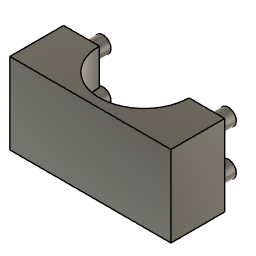
dpv2_cover (Autodesk Fusion 360 design; units mm, degrees)
Autodesk Fusion 360 part; units mm, degrees
note: some values were not read from the file. Set by a fixed rule: which face or edge a step refers to.
sketch "スケッチ1" plane through (0, 0, 0) normal (0, 1, 0) x (1, 0, 0)
  line L0 (-21, 0) -> (21, 0)
  line L1 (21, 0) -> (21, -72.5)
  line L2 (21, -72.5) -> (-21, -72.5)
  line L3 (-21, -72.5) -> (-21, 0)
  line L4 (6.5, -72.5) -> (-6.5, -72.5)
  line L5 (-6.5, -72.5) -> (-6.5, -96.5)
  line L6 (-6.5, -96.5) -> (6.5, -96.5)
  line L7 (6.5, -96.5) -> (6.5, -72.5)
  line L8 (-12.5, -160.5) -> (9, -160.5)
  line L9 (9, -160.5) -> (9, -96.5)
  line L10 (9, -96.5) -> (-12.5, -96.5)
  line L11 (-12.5, -96.5) -> (-12.5, -160.5)
  line L12 (-21, -67.5) -> (21, -67.5) construction
  circle A0 centre (-12, -67.5) radius 1.75
  circle A1 centre (12, -67.5) radius 1.75
  line L13 (0, -1.75) -> (0, -22.5)
  circle A2 centre (0, -155.5) radius 2
  dimension "d1" = 42
  dimension "d2" = 5
  dimension "d3" = 3.5
  dimension "d4" = 3.5
  dimension "d5" = 24
  dimension "d6" = 72.5
  dimension "d7" = 13
  dimension "d8" = 2.5
  dimension "d9" = 6
  dimension "d10" = 24
  dimension "d11" = 64
  dimension "d12" = 4
  dimension "d13" = 5
  constraint horizontal L0
  constraint vertical L1
  constraint horizontal L2
  constraint vertical L3
  constraint horizontal L4
  constraint vertical L5
  constraint horizontal L6
  constraint vertical L7
  constraint coincident L2 L4.start
  constraint horizontal L8
  constraint vertical L9
  constraint horizontal L10
  constraint vertical L11
  constraint midpoint origin L0
  constraint coincident L3 L12.start
  constraint coincident L1 L12.end
  constraint perpendicular L1 L12
  constraint coincident L12 A0.centre
  constraint coincident L12 A1.centre
  constraint symmetric A0 A1 L13
  constraint symmetric L5 L7 L13
  constraint coincident L13 A2.centre
  measures "d1" distance of L0.start L0.end
  measures "d2" distance of L2 L12
  measures "d3" diameter of A0
  measures "d4" diameter of A1
  measures "d5" distance of A0.centre A1.centre
  measures "d6" distance of L0.start L2.end
  measures "d7" distance of L5.end L6.end
  measures "d8" distance of L6.end L9.end
  measures "d9" distance of L5.end L10.end
  measures "d10" distance of L4.end L5.end
  measures "d11" distance of L8.start L10.end
  measures "d12" diameter of A2
  measures "d13" distance of L8 A2.centre
extrude "押し出し1" add sketch "スケッチ1" against normal blind 2 makes body 1
sketch "スケッチ2" plane through (0, 0, 0) normal (0, 1, 0) x (-1, 0, 0)
  circle A0 centre (12, 67.5) radius 1.75
  circle A1 centre (-12, 67.5) radius 1.75
  circle A2 centre (0, 155.5) radius 2
  line L0 (6.5, 72.5) -> (6.5, 96.5)
  line L1 (6.5, 96.5) -> (12.5, 96.5)
  line L2 (12.5, 96.5) -> (12.5, 160.5)
  line L3 (12.5, 160.5) -> (-9, 160.5)
  line L4 (-9, 160.5) -> (-9, 96.5)
  line L5 (-9, 96.5) -> (-6.5, 96.5)
  line L6 (-6.5, 96.5) -> (-6.5, 72.5)
  line L7 (-6.5, 72.5) -> (-21, 72.5)
  line L8 (-21, 72.5) -> (-21, 0)
  line L9 (-21, 0) -> (21, 0)
  line L10 (21, 0) -> (21, 72.5)
  line L11 (21, 72.5) -> (6.5, 72.5)
  line L12 (-21, 0) -> (-22.5, 0)
  line L13 (-22.5, 0) -> (-22.5, 74)
  line L14 (-22.5, 74) -> (-8, 74)
  line L15 (-8, 74) -> (-8, 95)
  line L16 (-8, 95) -> (-10.5, 95)
  line L17 (-10.5, 95) -> (-10.5, 160.5)
  line L18 (-10.5, 160.5) -> (-9, 160.5)
  line L19 (12.5, 160.5) -> (14, 160.5)
  line L20 (14, 160.5) -> (14, 95)
  line L21 (14, 95) -> (8, 95)
  line L22 (8, 95) -> (8, 74)
  line L23 (8, 74) -> (22.5, 74)
  line L24 (22.5, 74) -> (22.5, 0)
  line L25 (22.5, 0) -> (21, 0)
  dimension "d16" = 1.5
  dimension "d17" = 1.5
  dimension "d18" = 1.5
  dimension "d19" = 1.5
  dimension "d20" = 1.5
  dimension "d22" = 1.5
  dimension "d23" = 1.5
  dimension "d24" = 1.5
  dimension "d25" = 1.5
  dimension "d26" = 1.5
  constraint coincident L8.end L9.start
  constraint perpendicular L8 L12
  constraint perpendicular L9 L13
  constraint perpendicular L13 L14
  constraint perpendicular L14 L15
  constraint perpendicular L15 L16
  constraint perpendicular L16 L17
  constraint coincident L3.end L4.start
  constraint coincident L2.end L3.start
  constraint perpendicular L2 L19
  constraint perpendicular L3 L20
  constraint perpendicular L0 L21
  constraint perpendicular L3 L22
  constraint perpendicular L0 L23
  constraint perpendicular L3 L24
  constraint coincident L9.end L10.start
  constraint perpendicular L24 L25
  constraint perpendicular L17 L18
  measures "d16" distance of L2.end L19.end
  measures "d17" distance of L17.end L3.end
  measures "d18" distance of L6 L15
  measures "d19" distance of L5 L16
  measures "d20" distance of L7 L14
  measures "d22" distance of L8.end L12.end
  measures "d23" distance of L24.end L9.end
  measures "d24" distance of L11 L23
  measures "d25" distance of L0 L22
  measures "d26" distance of L1 L21
extrude "押し出し2" add sketch "スケッチ2" against normal blind 15 contours L0 L1 L2 L10 L11 L19 L20 L21 L22 L23 L24 L25 | L4 L5 L6 L7 L8 L12 L13 L14 L15 L16 L17 L18 bodies 1
sketch "スケッチ3" plane through (0, -2, 0) normal (0, -1, 0) x (1, 0, 0)
  circle A0 centre (-12, 67.5) radius 1.75
  circle A1 centre (12, 67.5) radius 1.75
  circle A2 centre (0, 155.5) radius 2
  line L0 (-6.5, 96.5) -> (-6.5, 72.5)
  line L1 (-6.5, 72.5) -> (-21, 72.5)
  line L2 (-21, 72.5) -> (-21, 0)
  line L3 (-21, 0) -> (21, 0)
  line L4 (21, 0) -> (21, 72.5)
  line L5 (21, 72.5) -> (6.5, 72.5)
  line L6 (6.5, 72.5) -> (6.5, 96.5)
  line L7 (6.5, 96.5) -> (9, 96.5)
  line L8 (9, 96.5) -> (9, 160.5)
  line L9 (9, 160.5) -> (-12.5, 160.5)
  line L10 (-12.5, 160.5) -> (-12.5, 96.5)
  line L11 (-12.5, 96.5) -> (-6.5, 96.5)
  line L12 (-21, 0) -> (21, 0)
  line L13 (21, 0) -> (21, 10)
  line L14 (21, 10) -> (-21, 10)
  line L15 (-21, 10) -> (-21, 0)
  line L16 (-21, 12.6) -> (21, 12.6)
  line L17 (21, 12.6) -> (21, 22.6)
  line L18 (21, 22.6) -> (-21, 22.6)
  line L19 (-21, 22.6) -> (-21, 12.6)
  dimension "d29" = 10
  dimension "d30" = 10
  dimension "d31" = 2.6
  constraint horizontal L12
  constraint vertical L13
  constraint horizontal L14
  constraint vertical L15
  constraint coincident L4 L13.end
  constraint coincident L2.end L3.start
  constraint horizontal L16
  constraint vertical L17
  constraint horizontal L18
  constraint vertical L19
  constraint coincident L4 L17.end
  constraint coincident L2 L16.start
  measures "d29" distance of L2.end L14.end
  measures "d30" distance of L16.start L18.end
  measures "d31" distance of L14 L16
extrude "押し出し3" add sketch "スケッチ3" along normal up to surface (13 mm away) contours L2 L4 L16 L17 L18 L19 | L2 L3 L4 L12 L13 L14 L15 bodies 1
sketch "スケッチ4" plane through (0, 0, 0) normal (0, 0, -1) x (1, 0, 0)
  line L0 (-22.5, 0) -> (22.5, 0)
  line L1 (22.5, 0) -> (22.5, 15)
  line L2 (22.5, 15) -> (-22.5, 15)
  line L3 (-22.5, 15) -> (-22.5, 0)
  arc A0 (-12.5, 15) -> (12.5, 15) centre (0, 15) ccw
  dimension "d34" = 25
  constraint midpoint L2 A0.centre
  constraint coincident L2 A0.end
  constraint coincident L2 A0.start
  measures "d34" diameter of A0
extrude "押し出し4" cut sketch "スケッチ4" against normal up to surface (22.6 mm away) contours L2 A0 bodies 1
sketch "スケッチ10" plane through (0, -2, 0) normal (0, -1, 0) x (1, 0, 0)
  circle A0 centre (12, 67.5) radius 1.75
  circle A1 centre (0, 155.5) radius 2
  circle A2 centre (-12, 67.5) radius 1.75
  line L0 (-21, 22.6) -> (21, 22.6)
  line L1 (21, 22.6) -> (21, 72.5)
  line L2 (21, 72.5) -> (6.5, 72.5)
  line L3 (6.5, 72.5) -> (6.5, 96.5)
  line L4 (6.5, 96.5) -> (9, 96.5)
  line L5 (9, 96.5) -> (9, 160.5)
  line L6 (9, 160.5) -> (-12.5, 160.5)
  line L7 (-12.5, 160.5) -> (-12.5, 96.5)
  line L8 (-12.5, 96.5) -> (-6.5, 96.5)
  line L9 (-6.5, 96.5) -> (-6.5, 72.5)
  line L10 (-6.5, 72.5) -> (-21, 72.5)
  line L11 (-21, 72.5) -> (-21, 22.6)
  circle A3 centre (0, 155.5) radius 4
  dimension "d48" = 8
  constraint concentric A1 A3
  measures "d48" diameter of A3
extrude "押し出し9" add sketch "スケッチ10" along normal blind 6 contours A3 bodies 1
sketch "スケッチ9" plane through (0, -2, 0) normal (0, -1, 0) x (1, 0, 0)
  circle A0 centre (12, 67.5) radius 1.75
  circle A1 centre (-12, 67.5) radius 1.75
  line L0 (-21, 22.6) -> (21, 22.6)
  line L1 (21, 22.6) -> (21, 72.5)
  line L2 (21, 72.5) -> (6.5, 72.5)
  line L3 (6.5, 72.5) -> (6.5, 96.5)
  line L4 (6.5, 96.5) -> (9, 96.5)
  line L5 (9, 96.5) -> (9, 160.5)
  line L6 (9, 160.5) -> (-12.5, 160.5)
  line L7 (-12.5, 160.5) -> (-12.5, 96.5)
  line L8 (-12.5, 96.5) -> (-6.5, 96.5)
  line L9 (-6.5, 96.5) -> (-6.5, 72.5)
  line L10 (-6.5, 72.5) -> (-21, 72.5)
  line L11 (-21, 72.5) -> (-21, 22.6)
  line L12 (-21, 72.5) -> (21, 72.5)
  line L13 (21, 72.5) -> (21, 62.5)
  line L14 (21, 62.5) -> (-21, 62.5)
  line L15 (-21, 62.5) -> (-21, 72.5)
  circle A2 centre (0, 155.5) radius 4
  dimension "d45" = 10
  constraint horizontal L12
  constraint vertical L13
  constraint horizontal L14
  constraint vertical L15
  constraint coincident L1 L13.end
  constraint coincident L10.end L11.start
  measures "d45" distance of L12 L14
extrude "押し出し8" add sketch "スケッチ9" along normal blind 1 contours L1 L2 L10 L11 L12 L13 L14 L15 bodies 1
ref_plane "作業平面1" through (0, -20, 80.25) normal (0, -1, 0) x (0, 0, -1)
sketch "スケッチ6" plane through (0, -20, 0) normal (0, -1, 0) x (-1, 0, 0)
  line L0 (-22.5, 0) -> (22.5, 0)
  line L1 (22.5, 0) -> (22.5, -22.6)
  line L2 (22.5, -22.6) -> (-22.5, -22.6)
  line L3 (-22.5, -22.6) -> (-22.5, 0)
  line L4 (-22.5, 0) -> (-22.5, -74)
  line L5 (-12.5, -22.6) -> (-21, -22.6)
  line L6 (-12.5, 0) -> (-22.5, 0)
  line L7 (22.5, -74) -> (22.5, 0)
  constraint horizontal L0
  constraint vertical L1
  constraint horizontal L2
  constraint vertical L3
  constraint collinear L3 L4
  constraint collinear L2 L5
  constraint collinear L0 L6
  constraint collinear L1 L7
extrude "押し出し5" add sketch "スケッチ6" along normal blind 15 separate body makes body 2
sketch "スケッチ7" plane through (0, 0, 0) normal (0, 0, -1) x (1, 0, 0)
  line L0 (-22.5, 20) -> (22.5, 20)
  line L1 (22.5, 20) -> (22.5, 35)
  line L2 (22.5, 35) -> (-22.5, 35)
  line L3 (-22.5, 35) -> (-22.5, 20)
  arc A0 (12.5, 20) -> (-12.5, 20) centre (0, 20) ccw
  dimension "d40" = 25
  constraint midpoint L0 A0.centre
  constraint coincident L0 A0.end
  constraint coincident L0 A0.start
  measures "d40" diameter of A0
extrude "押し出し6" cut sketch "スケッチ7" against normal up to surface (22.6 mm away) contours L0 A0 bodies 2
sketch "スケッチ8" plane through (0, -20, 0) normal (0, 1, 0) x (-1, 0, 0)
  line L0 (-12.5, 0) -> (-12.5, 22.6)
  line L1 (-12.5, 22.6) -> (-22.5, 22.6)
  line L2 (-22.5, 22.6) -> (-22.5, 0)
  line L3 (-22.5, 0) -> (-12.5, 0)
  line L4 (21, 12.6) -> (-21, 12.6)
  line L5 (-21, 12.6) -> (-21, 10)
  line L6 (-21, 10) -> (21, 10)
  line L7 (21, 10) -> (21, 12.6)
  point P0 (21, 12.6)
  point P1 (21, 10)
  point P2 (-21, 12.6)
  constraint horizontal L4
  constraint vertical L5
  constraint horizontal L6
  constraint vertical L7
  constraint coincident P0 L4.start
  constraint coincident P1 L6.end
  constraint coincident P2 L4.end
extrude "押し出し7" cut sketch "スケッチ8" against normal blind 13 contours L0 L4 L5 L6 | L0 L4 L6 L7 bodies 2
sketch "スケッチ11" plane through (0, -15, 0) normal (0, -1, 0) x (1, 0, 0)
  line L0 (-12.5, 0) -> (-12.5, 10)
  line L1 (-12.5, 10) -> (-21, 10)
  line L2 (-21, 10) -> (-21, 12.6)
  line L3 (-21, 12.6) -> (-12.5, 12.6)
  line L4 (-12.5, 12.6) -> (-12.5, 22.6)
  line L5 (-12.5, 22.6) -> (-21, 22.6)
  line L6 (-21, 22.6) -> (-21, 72.5)
  line L7 (-21, 72.5) -> (-6.5, 72.5)
  line L8 (-6.5, 72.5) -> (-6.5, 96.5)
  line L9 (-6.5, 96.5) -> (-12.5, 96.5)
  line L10 (-12.5, 96.5) -> (-12.5, 160.5)
  line L11 (-12.5, 160.5) -> (-14, 160.5)
  line L12 (-14, 160.5) -> (-14, 95)
  line L13 (-14, 95) -> (-8, 95)
  line L14 (-8, 95) -> (-8, 74)
  line L15 (-8, 74) -> (-22.5, 74)
  line L16 (-22.5, 74) -> (-22.5, 0)
  line L17 (-22.5, 0) -> (-12.5, 0)
  line L18 (-17.5, 17.6) -> (17.5, 17.6) construction
  line L19 (17.5, 17.6) -> (17.5, 5) construction
  line L20 (17.5, 5) -> (-17.5, 5) construction
  line L21 (-17.5, 5) -> (-17.5, 17.6) construction
  line L22 (22.5, 0) -> (22.5, 74)
  circle A0 centre (-17.5, 17.6) radius 2.5
  circle A1 centre (17.5, 17.6) radius 2.5
  circle A2 centre (-17.5, 5) radius 2.5
  circle A3 centre (17.5, 5) radius 2.5
  dimension "d51" = 5
  dimension "d52" = 5
  dimension "d53" = 5
  dimension "d54" = 5
  dimension "d55" = 5
  dimension "d56" = 5
  dimension "d57" = 5
  dimension "d58" = 5
  constraint horizontal L18
  constraint vertical L19
  constraint horizontal L20
  constraint vertical L21
  constraint coincident L18.start L21.end
  constraint coincident L18.end L19.start
  constraint coincident L20.end L21.start
  constraint coincident L19.end L20.start
  measures "d51" distance of L5 L18
  measures "d52" distance of L17 L20
  measures "d53" distance of L16 L21
  measures "d54" distance of L19 L22
  measures "d55" diameter of A0
  measures "d56" diameter of A1
  measures "d57" diameter of A2
  measures "d58" diameter of A3
extrude "押し出し10" cut sketch "スケッチ11" against normal blind 10 contours A0 | A1 | A2 | A3 bodies 1
sketch "スケッチ12" plane through (0, -20, 0) normal (0, 1, 0) x (-1, 0, 0)
  line L0 (12.5, 12.6) -> (21, 12.6)
  line L1 (21, 12.6) -> (21, 10)
  line L2 (21, 10) -> (12.5, 10)
  line L3 (12.5, 10) -> (12.5, 0)
  line L4 (12.5, 0) -> (22.5, 0)
  line L5 (22.5, 0) -> (22.5, 22.6)
  line L6 (22.5, 22.6) -> (12.5, 22.6)
  line L7 (12.5, 22.6) -> (12.5, 12.6)
  circle A0 centre (17.5, 17.6) radius 2.5
  circle A1 centre (17.5, 17.6) radius 2.5
  circle A2 centre (17.5, 5) radius 2.5
  circle A3 centre (-17.5, 17.6) radius 2.5
  circle A4 centre (-17.5, 5) radius 2.5
  circle A5 centre (-17.5, 17.6) radius 2.25
  circle A6 centre (-17.5, 5) radius 2.25
  circle A7 centre (17.5, 17.6) radius 2.25
  circle A8 centre (17.5, 5) radius 2.25
  dimension "d63" = 4.5
  dimension "d64" = 4.5
  dimension "d65" = 4.5
  dimension "d66" = 4.5
  constraint concentric A3 A5
  constraint concentric A4 A6
  constraint concentric A0 A7
  constraint concentric A2 A8
  measures "d63" diameter of A5
  measures "d64" diameter of A6
  measures "d65" diameter of A7
  measures "d66" diameter of A8
extrude "押し出し12" add sketch "スケッチ12" along normal blind 6 contours A5 | A6 | A7 | A8 bodies 2
sketch "スケッチ14" plane through (0, 0, 0) normal (0, 1, 0) x (-1, 0, 0)
  circle A0 centre (0, 155.5) radius 2
  circle A1 centre (12, 67.5) radius 1.75
  circle A2 centre (-12, 67.5) radius 1.75
  line L0 (14, 160.5) -> (-10.5, 160.5)
  line L1 (-10.5, 160.5) -> (-10.5, 95)
  line L2 (-10.5, 95) -> (-8, 95)
  line L3 (-8, 95) -> (-8, 74)
  line L4 (-8, 74) -> (-22.5, 74)
  line L5 (-22.5, 74) -> (-22.5, 0)
  line L6 (-22.5, 0) -> (22.5, 0)
  line L7 (22.5, 0) -> (22.5, 74)
  line L8 (22.5, 74) -> (8, 74)
  line L9 (8, 74) -> (8, 95)
  line L10 (8, 95) -> (14, 95)
  line L11 (14, 95) -> (14, 160.5)
  line L12 (14, 149) -> (15.5, 149)
  line L13 (15.5, 149) -> (14, 150.5)
  line L14 (14, 126.5) -> (15.5, 126.5)
  line L15 (15.5, 126.5) -> (14, 125)
  line L16 (-10.5, 150.5) -> (-12, 149)
  line L17 (-12, 149) -> (-10.5, 149)
  line L18 (-10.5, 126.5) -> (-12, 126.5)
  line L19 (-12, 126.5) -> (-10.5, 125)
  dimension "d79" = 10
  dimension "d80" = 10
  dimension "d81" = 1.5
  dimension "d82" = 1.5
  dimension "d83" = 22.5
  dimension "d84" = 1.5
  dimension "d85" = 1.5
  dimension "d86" = 1.5
  dimension "d88" = 1.5
  dimension "d89" = 1.5
  constraint coincident L11 L12.start
  constraint perpendicular L11 L12
  constraint coincident L11 L13.end
  constraint coincident L11 L14.start
  constraint perpendicular L11 L14
  constraint coincident L11 L15.end
  constraint coincident L1 L16.start
  constraint coincident L1 L17.end
  constraint perpendicular L1 L17
  constraint coincident L1 L18.start
  constraint perpendicular L1 L18
  constraint coincident L1 L19.end
  constraint collinear L12 L17
  constraint collinear L14 L18
  measures "d79" distance of L0.start L13.end
  measures "d80" distance of L0.end L16.start
  measures "d81" distance of L12.start L13.end
  measures "d82" distance of L12.start L12.end
  measures "d83" distance of L12.start L14.start
  measures "d84" distance of L14.start L14.end
  measures "d85" distance of L14.start L15.end
  measures "d86" distance of L16.end L17.end
  measures "d88" distance of L18.start L18.end
  measures "d89" distance of L18.start L19.end
extrude "押し出し13" add sketch "スケッチ14" against normal up to surface (15 mm away) contours L11 L12 L13 | L1 L16 L17 | L11 L14 L15 | L1 L18 L19 bodies 1
hidden bodies 1
